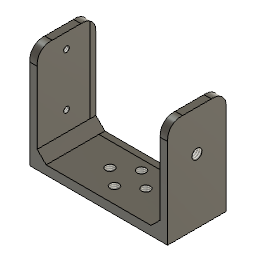
tiltrotormount (Autodesk Fusion 360 design; units mm, degrees)
part number: 2026-02-15-15-55-47-245
part number: 2026-02-15-15-56-22-795
Autodesk Fusion 360 part; units mm, degrees
sketch "Sketch1" plane through (0, 0, 0) normal (0, 0, 1) x (1, 0, 0) in component "Component"
  line L0 (-50, 30) -> (-50, 14.4)
  line L1 (-50, 14.4) -> (-5, 14.4)
  line L2 (-5, 14.4) -> (-5, 30)
  line L3 (-5, 30) -> (-50, 30)
  dimension "d1" = 15.6
  dimension "d2" = 45
  constraint perpendicular L0 L1
  constraint parallel L0 L2
  constraint parallel L1 L3
  constraint vertical L0
  measures "d1" distance of L0.start L0.end
  measures "d2" distance of L0.start L2.end
extrude "Extrude1" add sketch "Sketch1" along normal blind 2 in component "Component"
sketch "Sketch2" plane through (0, 0, 2) normal (0, 0, 1) x (-1, 0, 0) in component "Component"
  line L0 (5, -30) -> (50, -30)
  line L1 (50, -30) -> (50, -14.4)
  line L2 (50, -14.4) -> (5, -14.4)
  line L3 (5, -14.4) -> (5, -30)
  line L4 (50, -30) -> (50, -14.4)
  line L5 (50, -14.4) -> (48, -14.4)
  line L6 (48, -14.4) -> (48, -30)
  line L7 (48, -30) -> (50, -30)
  line L8 (5, -30) -> (5, -14.4)
  line L9 (5, -14.4) -> (7, -14.4)
  line L10 (7, -14.4) -> (7, -30)
  line L11 (7, -30) -> (5, -30)
  dimension "d5" = 2
  dimension "d6" = 2
  constraint perpendicular L4 L5
  constraint parallel L4 L6
  constraint parallel L5 L7
  constraint coincident L1.end L2.start
  constraint perpendicular L2 L4
  constraint coincident L0.end L1.start
  constraint perpendicular L8 L9
  constraint parallel L8 L10
  constraint parallel L9 L11
  constraint coincident L2.end L3.start
  constraint perpendicular L2 L8
  constraint coincident L0.start L3.end
  measures "d5" distance of L0.end L6.end
  measures "d6" distance of L0.start L10.end
sketch "Sketch3" plane through (0, 0, 2) normal (0, 0, 1) x (-1, 0, 0) in component "Component"
extrude "Extrude2" add sketch "Sketch2" along normal blind 32 contours L0 L2 L3 L8 L9 L10 L11 | L0 L1 L2 L4 L5 L6 L7 in component "Component"
sketch "Sketch4" plane through (-5, 0, 0) normal (1, 0, 0) x (0, 1, 0) in component "Component"
  line L0 (14.4, 0) -> (30, 0)
  line L1 (30, 0) -> (30, 34)
  line L2 (30, 34) -> (14.4, 34)
  line L3 (14.4, 34) -> (14.4, 0)
  line L4 (22.2004, 34) -> (22.2004, 20.5)
  dimension "d9" = 13.5
  constraint coincident L2 L4.start
  constraint perpendicular L2 L4
  measures "d9" distance of L4.start L4.end
sketch "Sketch5" plane through (-5, 0, 0) normal (1, 0, 0) x (0, 1, 0) in component "Component"
  line L0 (14.4, 34) -> (22.2, 34)
  dimension "d10" = 7.8
  constraint horizontal L0
  measures "d10" distance of L0.start L0.end
hole "Hole1" at (-5, 22.2004, 20.5) direction (-1, 0, 0) diameter 3.332 depth 2 tip angle 180 in component "Component"
thread "Thread1" "ISO Metric profile 4.0 M4x0.7 M4x0.7 6H" thread offset 0 thread depth 7.4 in component "Component"
sketch "Sketch6" plane through (-50, 0, 0) normal (-1, 0, 0) x (0, -1, 0) in component "Component"
  line L0 (-30, 0) -> (-14.4, 0)
  line L1 (-14.4, 0) -> (-14.4, 34)
  line L2 (-14.4, 34) -> (-30, 34)
  line L3 (-30, 34) -> (-30, 0)
  line L4 (-30, 34) -> (-22.2, 34)
  line L5 (-22.2, 34) -> (-22.2, 29)
  line L6 (-22.2, 29) -> (-22.2, 11.5)
  dimension "d16" = 7.8
  dimension "d17" = 5
  dimension "d18" = 17.5
  constraint coincident L2.end L3.start
  constraint perpendicular L3 L4
  constraint perpendicular L2 L5
  constraint parallel L5 L6
  measures "d16" distance of L2.end L4.end
  measures "d17" distance of L4.end L5.end
  measures "d18" distance of L5.end L6.end
hole "Hole2" at (-50, 22.2, 29) at (-50, 22.2, 11.5) direction (1, 0, 0) diameter 1.875 depth 5 tip angle 180 in component "Component"
thread "Thread2" "ISO Metric profile 2.3 M2.3x0.45 M2.3x0.45 6H" thread offset 0 thread depth 7.4 in component "Component"
sketch "Sketch7" plane through (-50, 0, 0) normal (-1, 0, 0) x (0, -1, 0) in component "Component"
  circle A0 centre (-22.2, 29) radius 0.9377
  circle A1 centre (-22.2, 11.5) radius 0.9377
  line L0 (-30, 0) -> (-14.4, 0)
  line L1 (-14.4, 0) -> (-14.4, 34)
  line L2 (-14.4, 34) -> (-30, 34)
  line L3 (-30, 34) -> (-30, 0)
  arc A2 (-14.4, 29) -> (-30, 29) centre (-22.2, 25.416) ccw
  constraint coincident L1 A2.start
  constraint coincident L3 A2.end
extrude "Extrude4" add 1 faces at (-5, 22.2001, 6.278) along direction (1, 0, 0) blind 0.5 in component "Component"
extrude "Extrude5" add 1 faces at (-50, 22.2, 3.5208) along direction (-1, 0, 0) blind 0.5 in component "Component"
sketch "Sketch8" plane through (0, 0, 0) normal (0, 1, 0) x (1, 0, 0) in component "Component"
sketch "Sketch9" plane through (0, 14.4, 0) normal (0, -1, 0) x (1, 0, 0) in component "Component"
  line L0 (-50.5, 34) -> (-50.5, 0)
  line L1 (-50.5, 0) -> (-4.5, 0)
  line L2 (-4.5, 0) -> (-4.5, 34)
  line L3 (-7, 34) -> (-7, 2)
  line L4 (-7, 2) -> (-48, 2)
  line L5 (-48, 2) -> (-48, 34)
  line L6 (-48, 5) -> (-45, 2)
  line L7 (-7, 5) -> (-10, 2)
  line L8 (-4.5, 34) -> (-7, 34)
  line L9 (-48, 34) -> (-50.5, 34)
  constraint coincident L5 L6.start
  constraint coincident L4 L6.end
  constraint coincident L3 L7.start
  constraint coincident L4 L7.end
  constraint perpendicular L6 L7
extrude "Extrude6" add sketch "Sketch9" against normal blind 15.6 contours L4 L5 L6 | L3 L4 L7 in component "Component"
sketch "Sketch10" plane through (0, 30, 0) normal (0, 1, 0) x (-1, 0, 0) in component "Component"
  line L0 (48, 34) -> (48, 5)
  line L1 (48, 5) -> (45, 2)
  line L2 (45, 2) -> (10, 2)
  line L3 (10, 2) -> (7, 5)
  line L4 (7, 5) -> (7, 34)
  line L5 (4.5, 34) -> (4.5, 0)
  line L6 (4.5, 0) -> (50.5, 0)
  line L7 (50.5, 0) -> (50.5, 34)
  line L8 (4.5, 0) -> (27, 0)
  line L9 (50.5, 34) -> (48, 34)
  line L10 (7, 34) -> (4.5, 34)
  dimension "d34" = 22.5
  constraint coincident L5.end L6.start
  constraint perpendicular L5 L8
  measures "d34" distance of L5.end L8.end
sketch "Sketch11" plane through (0, 30, 0) normal (0, 1, 0) x (-1, 0, 0) in component "Component"
extrude "Extrude7" add sketch "Sketch10" along normal blind 2 in component "Component"
extrude "Extrude8" add 1 faces at (-7.1667, 14.4, 2.3333) along direction (0, -1, 0) blind 2 in component "Component"
fillet "Fillet2" radius 5 curvature continuous 4 edges at (-5.75, 32, 34) (-49.25, 32, 34) (-49.25, 12.4, 34) (-5.75, 12.4, 34) in component "Component"
extrude "Extrude9" add 1 faces at (-35.1667, 18.9333, 0) along direction (0, 0, -1) blind 1 in component "Component"
sketch "Sketch12" plane through (0, 0, -1) normal (0, 0, -1) x (1, 0, 0) in component "Component"
  line L0 (-4.5, -32) -> (-4.5, -12.4)
  line L1 (-4.5, -12.4) -> (-50.5, -12.4)
  line L2 (-50.5, -12.4) -> (-50.5, -32)
  line L3 (-50.5, -32) -> (-4.5, -32)
  line L4 (-50.5, -32) -> (-50.5, -22.2)
  line L5 (-50.5, -12.4) -> (-27.5, -12.4)
  line L6 (-27.5, -12.4) -> (-27.5, -32)
  line L7 (-50.5, -22.2) -> (-27.5, -22.2)
  dimension "d43" = 9.8
  dimension "d44" = 23
  constraint coincident L2.end L3.start
  constraint perpendicular L3 L4
  constraint coincident L1.end L2.start
  constraint perpendicular L2 L5
  constraint midpoint L3 L6.end
  constraint midpoint L6 L7.end
  measures "d43" distance of L2.end L4.end
  measures "d44" distance of L1.end L5.end
sketch "Sketch13" plane through (0, 0, -1) normal (0, 0, -1) x (1, 0, 0) in component "Component"
  circle A0 centre (-27.5, -22.2) radius 8.5
  line L0 (-27.5, -22.2, 0) -> (-27.5, -22.2, 18.3755)
  dimension "d45" = 17
  measures "d45" diameter of A0
sketch "Sketch14" plane through (0, 0, -1) normal (0, 0, -1) x (1, 0, 0) in component "Component"
  line L0 (-27.5501, -22.1995) -> (-4.5501, -22.1995)
  dimension "d51" = 23
  constraint horizontal L0
  measures "d51" distance of L0.start L0.end
sketch "Sketch15" plane through (0, 0, -1) normal (0, 0, -1) x (1, 0, 0) in component "Component"
  line L0 (-27.5, -22.2) -> (-27.5, -17.7)
  line L1 (-27.5, -22.2) -> (-27.5, -26.7)
  line L2 (-27.5, -22.2) -> (-21.5, -22.2)
  line L3 (-27.5, -22.2) -> (-33.5, -22.2)
  dimension "d64" = 4.5
  dimension "d65" = 4.5
  dimension "d66" = 6
  dimension "d67" = 6
  constraint vertical L0
  constraint parallel L0 L1
  constraint perpendicular L0 L2
  constraint perpendicular L0 L3
  measures "d64" distance of L0.start L0.end
  measures "d65" distance of L0.start L1.end
  measures "d66" distance of L0.start L2.end
  measures "d67" distance of L0.start L3.end
hole "Hole8" at (-27.5, 17.7, -1) at (-27.5, 26.7, -1) at (-21.5, 22.2, -1) at (-33.5, 22.2, -1) direction (0, 0, 1) diameter 2.93 depth 5 tip angle 118 in component "Component"
thread "Thread8" "ISO Metric profile 3.5 M3.5x0.6 M3.5x0.6 6H" thread offset 0 thread depth 7.4 in component "Component"
sketch "Sketch1 (2)" plane through (0, 0, -1) normal (0, 0, -1) x (1, 0, 0)
  circle A0 centre (-27.5, -17.7) radius 0.9377
  circle A1 centre (-27.5, -26.7) radius 0.9377
  line L0 (-4.5, -32) -> (-4.5, -12.4)
  line L1 (-4.5, -12.4) -> (-50.5, -12.4)
  line L2 (-50.5, -12.4) -> (-50.5, -32)
  line L3 (-50.5, -32) -> (-4.5, -32)
  line L4 (-21.5, -22.2) -> (-19.5, -22.2)
  line L5 (-33.5, -22.2) -> (-35.5, -22.2)
  line L6 (-27.5, -17.7) -> (-27.5, -17.45)
  line L7 (-27.5, -26.7) -> (-27.5, -26.95)
  dimension "d80" = 2
  dimension "d81" = 0.25
  dimension "d82" = 0.25
  constraint horizontal L4
  constraint horizontal L5
  constraint coincident A0.centre L6.start
  constraint vertical L6
  constraint coincident A1.centre L7.start
  constraint vertical L7
  measures "d80" distance of L5.start L5.end
  measures "d81" distance of A0.centre L6.end
  measures "d82" distance of A1.centre L7.end
sketch "Sketch16" plane through (0, 0, -1) normal (0, 0, -1) x (1, 0, 0) in component "Component"
  circle A0 centre (-27.5, -17.7) radius 0.9377
  circle A1 centre (-27.5, -26.7) radius 0.9377
  line L0 (-4.5, -32) -> (-4.5, -12.4)
  line L1 (-4.5, -12.4) -> (-50.5, -12.4)
  line L2 (-50.5, -12.4) -> (-50.5, -32)
  line L3 (-50.5, -32) -> (-4.5, -32)
  line L4 (-27.5, -22.2) -> (-23, -22.2)
  line L5 (-27.5, -22.2) -> (-32, -22.2)
  dimension "d73" = 4.5
  dimension "d74" = 4.5
  constraint parallel L1 L4
  constraint parallel L4 L5
  measures "d73" distance of L4.start L4.end
  measures "d74" distance of L4.start L5.end
component "Component" placed x (1, 0, 0) y (0, 1, 0) z (0, 0, 1) at (0, 0, 0)
